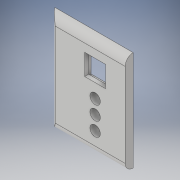
# Autodesk Inventor part: Case Front
Saved by Autodesk Inventor 2019 (Build 230136000, 136)
## iProperties
Created: 2022-04-25
Part Number: Case Front
Material: Generic
Document SubType Name: Modeling
Designer: Loxei
Density: 1 g/cm^3
Appearance: Default
Author: Loxei
Autodesk Inventor part; units mm, degrees
ref_plane "YZ Plane" through (0, 0, 0) normal (1, 0, 0) x (0, 1, 0)
ref_plane "XZ Plane" through (0, 0, 0) normal (0, 1, 0) x (-1, 0, 0)
ref_plane "XY Plane" through (0, 0, 0) normal (0, 0, 1) x (1, 0, 0)
sketch "Sketch1" plane through (0, 0, 0) normal (0, 1, 0) x (-1, 0, 0)
  line L0 (0, 65.172) -> (0, -65.172) construction
  line L1 (43.74, 0) -> (-43.74, 0) construction
  spline S0 degree 3 poles (-5.8666, 35) (13.8832, 21.2522) (-10.0462, -16.0043) (8.551, -35) knots 1 1 1 1 2 2 2 2
  line L2 (-5.8666, 35) -> (13.8832, 21.2522) construction
  line L3 (13.8832, 21.2522) -> (-10.0462, -16.0043) construction
  line L4 (-10.0462, -16.0043) -> (8.551, -35) construction
  line L5 (-5.8666, 35) -> (-40.8666, 35)
  line L6 (-1.7165, 31) -> (-40.8666, 31)
  line L7 (-40.8666, 35) -> (-40.8666, 31)
  point P0 (0, 0)
  point P1 (0, 0)
  point P2 (0, 0)
  point P3 (0, 0)
  dimension "d0" = 35
  dimension "d1" = 4
  constraints: 10 end point, 4 midpoint, 2 perpendicular, 2 symmetric about line, 2 vertical, 1 coincident, 1 horizontal, 1 parallel, 4 other
  measures "d0" distance of L2.start L5.end
  measures "d1" distance between parallel lines of L5 L6
extrude "Extrusion1" add sketch "Sketch1" along normal blind 50
fillet "Fillet1" radius 4 2 edges at (23.3666, 50, 35) (23.3666, 0, 35)
sketch "Sketch2" plane through (5.8666, 4, 35) normal (0, 0, 1) x (1, 0, 0)
  circle A0 centre (20, 6.6) radius 2.6
  circle A1 centre (20, 13.5667) radius 2.6
  circle A2 centre (20, 20.5333) radius 2.6
  line L0 (14.75, 27.5) -> (25.25, 27.5)
  line L1 (25.25, 27.5) -> (25.25, 38)
  line L2 (25.25, 38) -> (14.75, 38)
  line L3 (14.75, 38) -> (14.75, 27.5)
  line L4 (35, 0) -> (35, 42) projected
  line L5 (35, 0) -> (0, 0) projected
  line L6 (0, 42) -> (35, 42) projected
  point P0 (-5.8666, -4)
  dimension "d5" = 5.2
  dimension "d6" = 5.2
  dimension "d7" = 5.2
  dimension "d8" = 10.5
  dimension "d9" = 10.5
  dimension "d10" = 15
  dimension "d11" = 15
  dimension "d12" = 15
  dimension "d13" = 6.6
  dimension "d14" = 4
  dimension "d15" = 6.9667
  dimension "d16" = 6.9667
  dimension "d17" = 6.9667
  dimension "d18" = 20.25
  constraints: 8 end point, 3 centre point, 2 parallel, 1 horizontal, 1 perpendicular
  measures "d5" diameter of A0
  measures "d6" diameter of A1
  measures "d7" diameter of A2
  measures "d8" distance of L2.end L0.start
  measures "d9" distance of L1.end L2.end
  measures "d10" distance from line of L4 A0.centre
  measures "d11" distance from line of L4 A1.centre
  measures "d12" distance from line of L4 A2.centre
  measures "d13" distance from line of L5 A0.centre
  measures "d14" distance between parallel lines of L6 L2
  measures "d15" distance of A1.centre A0.centre
  measures "d16" distance of A2.centre A1.centre
  measures "d17" distance from line of L0 A2.centre
  measures "d18" distance between parallel lines of L4 L3
extrude "Extrusion2" cut sketch "Sketch2" against normal blind 70
sketch "Sketch3" plane through (40.8666, 0, 31) normal (0, 0, -1) x (-1, 0, 0)
  line L0 (20.25, 31.5) -> (9.75, 31.5) projected
  line L1 (20.25, 42) -> (20.25, 31.5) projected
  line L2 (9.75, 31.5) -> (9.75, 42) projected
  line L3 (9.75, 42) -> (20.25, 42) projected
  line L4 (21.05, 43.3) -> (8.95, 43.3)
  line L5 (8.95, 43.3) -> (8.95, 30.2)
  line L6 (8.95, 30.2) -> (21.05, 30.2)
  line L7 (21.05, 30.2) -> (21.05, 43.3)
  line L8 (4.9766, 36.75) -> (25.0234, 36.75) construction
  line L9 (15, 47.4174) -> (15, 24.5333) construction
  circle A0 centre (15, 24.5333) radius 2.6 construction
  point P0 (40.8666, 0)
  point P1 (15, 36.75)
  dimension "d21" = 13.1
  dimension "d22" = 12.1
  dimension "d25" = 5.25
  dimension "d28" = 10.5
  constraints: 12 end point, 2 horizontal, 2 parallel, 2 perpendicular, 1 coincident, 1 midpoint, 1 point on line, 1 vertical, 2 other
  measures "d21" distance of L6.end L4.start
  measures "d22" distance of L5.end L6.end
  measures "d25" distance from line of L0 point (15, 36.75)
  measures "d28" distance between parallel lines of L0 L3
extrude "Extrusion3" cut sketch "Sketch3" against normal blind 2
equation "\"d6\" = d5"
equation "\"d7\" = d6"
equation "\"d9\" = d8"
equation "\"d11\" = d10"
equation "\"d12\" = d11"
equation "\"d13\" = d14 + 0.5 * d5"
equation "\"d15\" = d16"
equation "\"d16\" = d17"
equation "\"d18\" = d12 + 0.5 * d9"
equation "\"d25\" = 0.5 * d28"
body "Solid1"
